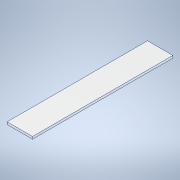
# Autodesk Inventor part: 與滑塊固定板金
Saved by Autodesk Inventor 2021 (Build 250183000, 183)
## iProperties
Created: 2023-01-12
Part Number: 與滑塊固定板金
Material: 鋁合金 6061
Document SubType Name: Sheet Metal
Designer: brian
Density: 2.7 g/cm^3
Appearance: 鋁 - 平面
Sheet Metal Rule: 預設
Author: brian
Autodesk Inventor part; units mm, degrees
ref_plane "YZ Plane" through (0, 0, 0) normal (1, 0, 0) x (0, 1, 0)
ref_plane "XZ Plane" through (0, 0, 0) normal (0, 1, 0) x (-1, 0, 0)
ref_plane "XY Plane" through (0, 0, 0) normal (0, 0, 1) x (1, 0, 0)
sketch "草圖1" plane through (0, 0, 0) normal (0, 1, 0) x (-1, 0, 0)
  line L0 (-16, 88.5) -> (16, 88.5)
  line L1 (16, 88.5) -> (16, -88.5)
  line L2 (16, -88.5) -> (-16, -88.5)
  line L3 (-16, -88.5) -> (-16, 88.5)
  line L4 (-16, 88.5) -> (16, -88.5) construction
  line L5 (16, 88.5) -> (-16, -88.5) construction
  point P0 (0, 0)
  dimension "d0" = 32
  dimension "d1" = 177
  constraints: 12 end point, 2 midpoint, 2 parallel, 1 horizontal, 1 perpendicular
  measures "d0" distance of L1.end L2.end
  measures "d1" distance of L0.end L1.end
extrude "擠出1" add sketch "草圖1" along normal blind 3
equation "\"折彎半徑\" = 厚度"
equation "\"折彎離隙寬度\" = 厚度"
equation "\"折彎離隙深度\" = 0.5 * 厚度"
equation "\"轉角離隙大小\" = 4 * 厚度"
equation "\"最小剩餘\" = 2 * 厚度"
equation "\"轉移半徑\" = 折彎半徑"
equation "\"Jacobi半徑大小\" = 厚度"
equation "\"間隙大小\" = 厚度"
equation "\"厚度\" = 0.5"
